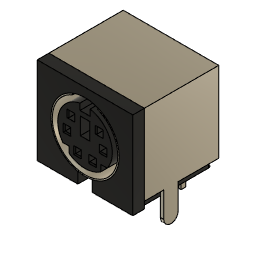
CUI_MD-60SM (Autodesk Fusion 360 design; units mm, degrees)
Autodesk Fusion 360 part; units mm, degrees
note: some values were not read from the file. Set by a fixed rule: which sketch regions a step uses.
sketch "Sketch1" plane through (0, 0, 0) normal (0, 1, 0) x (1, 0, 0) in component "Front"
  line L0 (-7, 0) -> (7, 0)
  line L1 (7, 0) -> (7, -12.8)
  line L2 (7, -12.8) -> (-7, -12.8)
  line L3 (-7, -12.8) -> (-7, 0)
  circle A0 centre (0, -6.5) radius 5
  line L4 (0, 0) -> (0, -12.8) construction
  dimension "d2" = 14
  dimension "d3" = 12.8
  dimension "d4" = 10
  dimension "d5" = 6.5
  constraint horizontal L0
  constraint vertical L1
  constraint horizontal L2
  constraint vertical L3
  constraint midpoint L4.start L0
  constraint coincident L4.start origin
  constraint midpoint L2 L4.end
  constraint coincident A0.centre L4
  measures "d2" distance of L0.start L0.end
  measures "d3" distance of L0.start L2.end
  measures "d4" diameter of A0
  measures "d5" distance of L4.start A0.centre
extrude "Extrude1" add sketch "Sketch1" along normal blind 1.7 makes body 1 in component "Front"
sketch "Sketch1 (2)" plane through (0, 1.7, 0) normal (0, 1, 0) x (-1, 0, 0) in component "Base"
  circle A0 centre (0, 6.5) radius 5
  line L0 (7, 12.8) -> (-7, 12.8)
  line L1 (-7, 12.8) -> (-7, 0)
  line L2 (-7, 0) -> (7, 0)
  line L3 (7, 0) -> (7, 12.8)
  line L4 (-6.5, 0) -> (6.5, 0)
  line L5 (6.5, 0) -> (6.5, 3.6)
  line L6 (6.5, 3.6) -> (-6.5, 3.6)
  line L7 (-6.5, 3.6) -> (-6.5, 0)
  dimension "d8" = 3.6
  dimension "d13" = 0.5
  constraint horizontal L4
  constraint vertical L5
  constraint horizontal L6
  constraint vertical L7
  constraint coincident L4.start L7.end
  constraint coincident L5.end L6.start
  constraint coincident L4.end L5.start
  constraint midpoint origin L4
  measures "d8" distance of L4.end L5.end
  measures "d13" distance of L1.end L4.start
extrude "Extrude1'" add sketch "Sketch1 (2)" along normal blind 10.4 separate body contours A0 L6 | A0 L2 L4 L5 L6 L7 picked at (-1.2021, 3.4122) makes body 2 in component "Base"
sketch "Sketch2" plane through (0, 1.7, 0) normal (0, -1, 0) x (1, 0, 0) in component "Base"
  line L0 (6.5, 0) -> (6.5, 3.6)
  line L1 (6.5, 3.6) -> (-6.5, 3.6)
  line L2 (-6.5, 3.6) -> (-6.5, 0)
  line L3 (-6.5, 0) -> (6.5, 0)
  circle A0 centre (0, 6.5) radius 5
extrude "Extrude2" cut sketch "Sketch2" against normal blind 3.3 contours L1 A0 | L1 A0 bodies 2 in component "Base"
fillet "Fillet1" radius 0.5 2 edges at (6.5, 12.1, 1.8) (-6.5, 12.1, 1.8) on bodies 2 in component "Base"
sketch "Sketch3" plane through (0, 0, 3.6) normal (0, 0, 1) x (-1, 0, 0) in component "Base"
  arc A0 (6, -12.1) -> (6.5, -11.6) centre (6, -11.6) ccw
  line L0 (6.5, -11.6) -> (6.5, -1.7)
  line L1 (6.5, -1.7) -> (4.0731, -1.7)
  line L2 (4.0731, -1.7) -> (4.0731, -5)
  line L3 (4.0731, -5) -> (-4.0731, -5)
  line L4 (-4.0731, -5) -> (-4.0731, -1.7)
  line L5 (-4.0731, -1.7) -> (-6.5, -1.7)
  line L6 (-6.5, -1.7) -> (-6.5, -11.6)
  arc A1 (-6.5, -11.6) -> (-6, -12.1) centre (-6, -11.6) ccw
  line L7 (-6, -12.1) -> (6, -12.1)
  line L8 (6.5, -5) -> (-6.5, -5)
  line L9 (-6.5, -5) -> (-6.5, -7)
  line L10 (-6.5, -7) -> (6.5, -7)
  line L11 (6.5, -7) -> (6.5, -5)
  dimension "d16" = 2
  constraint horizontal L8
  constraint vertical L9
  constraint horizontal L10
  constraint vertical L11
  constraint coincident L0 L8.start
  constraint collinear L6 L9
  constraint coincident L3.end L8
  measures "d16" distance of L8.start L10.end
extrude "Extrude3" add sketch "Sketch3" along normal up to surface (8.7 mm away) contours L0 L3 L6 L8 L9 L10 L11 bodies 2 in component "Base"
sketch "Sketch1 (3)" plane through (0, 5, 0) normal (0, -1, 0) x (1, 0, 0) in component "Jack"
  arc A0 (-4.0731, 3.6) -> (4.0731, 3.6) centre (0, 6.5) ccw
  line L0 (4.0731, 3.6) -> (6.5, 3.6)
  line L1 (6.5, 3.6) -> (6.5, 12.3)
  line L2 (6.5, 12.3) -> (-6.5, 12.3)
  line L3 (-6.5, 12.3) -> (-6.5, 3.6)
  line L4 (-6.5, 3.6) -> (-4.0731, 3.6)
  circle A1 centre (0, 6.5) radius 5
  circle A2 centre (0, 6.5) radius 4 construction
  line L5 (-0.75, 10.4291) -> (-0.75, 9.5)
  line L6 (-0.75, 9.5) -> (0.75, 9.5)
  line L7 (0.75, 9.5) -> (0.75, 10.4291)
  line L8 (0, 12.3) -> (0, 0) construction
  line L9 (-3.2524, 4.1716) -> (-2.3284, 4.1716)
  line L10 (-2.3284, 4.1716) -> (-2.3284, 3.2476)
  line L11 (3.2524, 4.1716) -> (2.3284, 4.1716)
  line L12 (2.3284, 4.1716) -> (2.3284, 3.2476)
  arc A3 (-0.75, 10.4291) -> (-3.2524, 4.1716) centre (0, 6.5) ccw
  arc A4 (3.2524, 4.1716) -> (0.75, 10.4291) centre (0, 6.5) ccw
  arc A5 (-2.3284, 3.2476) -> (2.3284, 3.2476) centre (0, 6.5) ccw
  dimension "d19" = 8
  dimension "d20" = 1.5
  dimension "d21" = 0.9291
  dimension "d22" = 0.924
  constraint concentric A0 A2
  constraint coincident A2 L5.start
  constraint vertical L5
  constraint perpendicular L5 L6
  constraint coincident A2 L7.end
  constraint perpendicular L6 L7
  constraint midpoint L2 L8.start
  constraint coincident L8.end origin
  constraint symmetric L5.end L6.end L8
  constraint coincident A2 L9.start
  constraint horizontal L9
  constraint coincident A2 L10.end
  constraint perpendicular L9 L10
  constraint coincident A2 L11.start
  constraint perpendicular L10 L11
  constraint coincident A2 L12.end
  constraint perpendicular L11 L12
  constraint equal L9 L10
  constraint equal L10 L11
  constraint equal L11 L12
  constraint concentric A2 A3
  constraint coincident A0.centre A1.centre
  constraint concentric A2 A4
  measures "d19" diameter of A2
  measures "d20" distance of L5.end L6.end
  measures "d21" distance of L6.end L7.end
  measures "d22" distance of L9.start L9.end
extrude "Extrude1''" add sketch "Sketch1 (3)" along normal up to surface (5 mm away) separate body contours L5 L6 L7 L9 L10 L11 L12 A3 A4 A5 makes body 3 in component "Jack"
sketch "Sketch2 (2)" plane through (0, 0, 0) normal (0, -1, 0) x (1, 0, 0) in component "Jack"
  line L0 (-0.75, 9.5) -> (-0.75, 10.4291)
  arc A0 (-0.75, 10.4291) -> (-3.2524, 4.1716) centre (0, 6.5) ccw
  line L1 (-3.2524, 4.1716) -> (-2.3284, 4.1716)
  line L2 (-2.3284, 4.1716) -> (-2.3284, 3.2476)
  arc A1 (-2.3284, 3.2476) -> (2.3284, 3.2476) centre (0, 6.5) ccw
  line L3 (2.3284, 3.2476) -> (2.3284, 4.1716)
  line L4 (2.3284, 4.1716) -> (3.2524, 4.1716)
  arc A2 (3.2524, 4.1716) -> (0.75, 10.4291) centre (0, 6.5) ccw
  line L5 (0.75, 10.4291) -> (0.75, 9.5)
  line L6 (0.75, 9.5) -> (-0.75, 9.5)
  circle A3 centre (0, 6.5) radius 4 construction
  line L7 (0, 0) -> (0, 12.3) construction
  line L8 (-4, 6.5) -> (4, 6.5) construction
  line L9 (-2.5, 8.585) -> (-1.65, 8.585)
  line L10 (-1.65, 8.585) -> (-1.65, 7.635)
  line L11 (-1.65, 7.635) -> (-2.5, 7.635)
  line L12 (-2.5, 7.635) -> (-2.5, 8.585)
  line L13 (1.65, 8.585) -> (2.5, 8.585)
  line L14 (2.5, 8.585) -> (2.5, 7.635)
  line L15 (2.5, 7.635) -> (1.65, 7.635)
  line L16 (1.65, 7.635) -> (1.65, 8.585)
  line L17 (-3.055, 6.515) -> (-2.105, 6.515)
  line L18 (-2.105, 6.515) -> (-2.105, 5.665)
  line L19 (-2.105, 5.665) -> (-3.055, 5.665)
  line L20 (-3.055, 5.665) -> (-3.055, 6.515)
  line L21 (2.105, 6.515) -> (3.055, 6.515)
  line L22 (3.055, 6.515) -> (3.055, 5.665)
  line L23 (3.055, 5.665) -> (2.105, 5.665)
  line L24 (2.105, 5.665) -> (2.105, 6.515)
  line L25 (-1.51, 4.435) -> (-0.56, 4.435)
  line L26 (-0.56, 4.435) -> (-0.56, 3.585)
  line L27 (-0.56, 3.585) -> (-1.51, 3.585)
  line L28 (-1.51, 3.585) -> (-1.51, 4.435)
  line L29 (0.56, 4.435) -> (1.51, 4.435)
  line L30 (1.51, 4.435) -> (1.51, 3.585)
  line L31 (1.51, 3.585) -> (0.56, 3.585)
  line L32 (0.56, 3.585) -> (0.56, 4.435)
  line L33 (2.105, 6.515) -> (3.055, 5.665) construction
  line L34 (3.055, 6.515) -> (2.105, 5.665) construction
  line L35 (1.65, 8.585) -> (2.5, 7.635) construction
  line L36 (2.5, 8.585) -> (1.65, 7.635) construction
  line L37 (-2.5, 8.585) -> (-1.65, 7.635) construction
  line L38 (-1.65, 8.585) -> (-2.5, 7.635) construction
  line L39 (-3.055, 6.515) -> (-2.105, 5.665) construction
  line L40 (-2.105, 6.515) -> (-3.055, 5.665) construction
  line L41 (-1.51, 4.435) -> (-0.56, 3.585) construction
  line L42 (-0.56, 4.435) -> (-0.4693, 4.435)
  line L43 (-1.51, 3.585) -> (-0.56, 4.435) construction
  line L44 (0.56, 4.435) -> (1.51, 3.585) construction
  line L45 (1.51, 4.435) -> (0.56, 3.585) construction
  line L46 (-2.075, 8.585) -> (-2.075, 7.635) construction
  line L47 (2.075, 8.585) -> (2.075, 7.635) construction
  line L48 (-2.075, 8.11) -> (2.075, 8.11) construction
  line L49 (-2.58, 6.515) -> (-2.58, 6.4)
  line L50 (-2.58, 6.4) -> (-2.58, 5.665) construction
  line L51 (2.58, 6.515) -> (2.58, 5.665) construction
  line L52 (-2.58, 6.09) -> (2.58, 6.09) construction
  line L53 (-1.035, 4.01) -> (1.035, 4.01) construction
  line L54 (0.69, 6.32) -> (-0.69, 6.32)
  line L55 (-0.69, 6.32) -> (-0.69, 8.81)
  line L56 (-0.69, 8.81) -> (0.69, 8.81)
  line L57 (0.69, 8.81) -> (0.69, 6.32)
  line L58 (0.69, 6.32) -> (-0.69, 8.81) construction
  line L59 (-0.69, 6.32) -> (0.69, 8.81) construction
  point P0 (0, 7.565)
  dimension "d27" = 0.85
  dimension "d28" = 0.95
  dimension "d29" = 0.85
  dimension "d30" = 0.95
  dimension "d43" = 5.16
  dimension "d48" = 8
  dimension "d49" = 4.15
  dimension "d50" = 2.07
  dimension "d51" = 1.61
  dimension "d52" = 0.41
  dimension "d53" = 2.49
  dimension "d54" = 1.38
  dimension "d55" = 2.49
  dimension "d56" = 2.31
  constraint tangent A0 A3
  constraint concentric A2 A3
  constraint coincident L7.start origin
  constraint vertical L7
  constraint coincident A3 L8.start
  constraint coincident A2 L8.end
  constraint coincident A0.centre L8
  constraint horizontal L8
  constraint horizontal L9
  constraint vertical L10
  constraint horizontal L11
  constraint vertical L12
  constraint horizontal L13
  constraint vertical L14
  constraint horizontal L15
  constraint vertical L16
  constraint horizontal L17
  constraint vertical L18
  constraint horizontal L19
  constraint vertical L20
  constraint horizontal L21
  constraint vertical L22
  constraint horizontal L23
  constraint vertical L24
  constraint horizontal L25
  constraint vertical L26
  constraint horizontal L27
  constraint vertical L28
  constraint horizontal L29
  constraint vertical L30
  constraint horizontal L31
  constraint vertical L32
  constraint equal L25 L29
  constraint equal L28 L32
  constraint equal L17 L25
  constraint equal L17 L21
  constraint equal L20 L28
  constraint equal L20 L24
  constraint equal L9 L13
  constraint equal L12 L16
  constraint collinear L19 L23
  constraint collinear L27 L31
  constraint coincident L25 L42.end
  constraint midpoint L9 L46.start
  constraint midpoint L11 L46.end
  constraint midpoint L13 L47.start
  constraint midpoint L15 L47.end
  constraint midpoint L46 L48.start
  constraint midpoint L36 L48.end
  constraint perpendicular L47 L48
  constraint symmetric L7 L48.start L48.end
  constraint midpoint L17 L49.start
  constraint perpendicular L17 L49
  constraint midpoint L19 L50.end
  constraint perpendicular L19 L50
  constraint midpoint L21 L51.start
  constraint midpoint L23 L51.end
  constraint midpoint L39 L52.start
  constraint midpoint L51 L52.end
  constraint perpendicular L51 L52
  constraint symmetric L7 L52.start L52.end
  constraint midpoint L41 L53.start
  constraint midpoint L44 L53.end
  constraint symmetric L7 L53.start L53.end
  constraint horizontal L54
  constraint perpendicular L54 L55
  constraint parallel L54 L56
  constraint parallel L55 L57
  constraint coincident L58 P0
  constraint coincident L59 P0
  constraint coincident L7 P0
  measures "d27" distance of L25.start L27.end
  measures "d28" distance of L25.start L25.end
  measures "d29" distance of L9.start L9.end
  measures "d30" distance of L9.start L11.end
  measures "d43" distance of L52.start L52.end
  measures "d48" diameter of A3
  measures "d49" distance of L48.start L48.end
  measures "d50" distance of L53.start L53.end
  measures "d51" distance of L8 L48
  measures "d52" distance of L8 L52
  measures "d53" distance of L8 L53
  measures "d54" distance of L55.end L56.end
  measures "d55" distance of L54.end L55.end
  measures "d56" distance of L8 L56.end
extrude "Extrude2'" cut sketch "Sketch2 (2)" against normal blind 5 contours L9 L10 L11 L12 | L13 L14 L15 L16 | L17 L18 L19 L20 | L21 L22 L23 L24 | L25 L26 L27 L28 | L29 L30 L31 L32 | L54 L55 L56 L57 bodies 3 in component "Jack"
chamfer "Chamfer1" distance 0.15 angle 45 18 edges at (-2.5, 0, 8.11) (-2.075, 0, 8.585) (-1.65, 0, 8.11) (1.65, 0, 8.11) (2.075, 0, 8.585) (2.5, 0, 8.11) (-2.58, 0, 6.515) (-3.055, 0, 6.09) (-2.58, 0, 5.665) (-1.035, 0, 4.435) (-1.51, 0, 4.01) (-1.035, 0, 3.585) (1.035, 0, 3.585) (1.51, 0, 4.01) (1.035, 0, 4.435) (2.58, 0, 5.665) (3.055, 0, 6.09) (2.58, 0, 6.515) on bodies 3 in component "Jack"
sketch "Sketch1 (4)" plane through (0, 5, 0) normal (0, -1, 0) x (1, 0, 0) in component "Barrel"
  arc A0 (-4.0731, 3.6) -> (4.0731, 3.6) centre (0, 6.5) ccw
  line L0 (4.0731, 3.6) -> (6.5, 3.6)
  line L1 (6.5, 3.6) -> (6.5, 12.3)
  line L2 (6.5, 12.3) -> (-6.5, 12.3)
  line L3 (-6.5, 12.3) -> (-6.5, 3.6)
  line L4 (-6.5, 3.6) -> (-4.0731, 3.6)
  circle A1 centre (0, 6.5) radius 5
  arc A2 (-1.9134, 11.1194) -> (1.9134, 11.1194) centre (0, 6.5) ccw
  line L5 (0, 6.5) -> (-1.9134, 11.1194) construction
  line L6 (0, 6.5) -> (1.9134, 11.1194) construction
  line L7 (0, 6.5) -> (0, 12.3) construction
  arc A3 (-1.8369, 10.9346) -> (1.8369, 10.9346) centre (0, 6.5) ccw
  line L8 (1.8369, 10.9346) -> (1.9134, 11.1194)
  line L9 (-1.8369, 10.9346) -> (-1.9134, 11.1194)
  dimension "d58" = 315
  dimension "d60" = 0.2
  constraint coincident A1 A2.start
  constraint coincident A0.centre A1.centre
  constraint midpoint L2 L7.end
  constraint symmetric A2.start A2.end L7
  constraint coincident L5 A3.start
  constraint parallel L6 L8
  measures "d60" distance of A2.end A3.end
extrude "Extrude1'''" add sketch "Sketch1 (4)" along normal up to surface (5 mm away) separate body contours A0 A1 A2 A3 L8 L9 makes body 4 in component "Barrel"
sketch "Sketch2 (3)" plane through (0, 0, 0) normal (0, -1, 0) x (1, 0, 0) in component "Front"
  circle A0 centre (0, 6.5) radius 5
  line L0 (7, 12.8) -> (-7, 12.8)
  line L1 (-7, 12.8) -> (-7, 0)
  line L2 (-7, 0) -> (7, 0)
  line L3 (7, 0) -> (7, 12.8)
  circle A1 centre (0, 6.5) radius 5
  line L4 (-7, 0) -> (7, 0)
  line L5 (0, 0) -> (0, 6.5) construction
  line L6 (1.05, 1.6115) -> (1.05, 0)
  line L7 (-1.05, 1.6115) -> (-1.05, 0)
  line L8 (-1.05, 0) -> (1.05, 0)
  dimension "d63" = 2.1
  constraint coincident L5.start origin
  constraint coincident A0.centre A1.centre
  constraint coincident A1 L6.start
  constraint coincident L2 L6.end
  constraint perpendicular L2 L6
  constraint coincident A1 L7.start
  constraint coincident L4 L7.end
  constraint perpendicular L4 L7
  constraint symmetric L5 L6.end L7.end
  measures "d63" distance of L6.end L7.end
extrude "Extrude2''" cut sketch "Sketch2 (3)" against normal up to surface (1.7 mm away) contours A0 L2 A1 L4 L6 L7 L8 bodies 1 in component "Front"
sketch "Sketch1 (5)" plane through (0, 1.7, 0) normal (0, 1, 0) x (-1, 0, 0) in component "Shield"
  line L0 (-1.05, 0) -> (-1.05, 1.6115)
  arc A0 (1.05, 1.6115) -> (-1.05, 1.6115) centre (0, 6.5) ccw
  line L1 (1.05, 1.6115) -> (1.05, 0)
  line L2 (1.05, 0) -> (7, 0)
  line L3 (7, 0) -> (7, 12.8)
  line L4 (7, 12.8) -> (-7, 12.8)
  line L5 (-7, 12.8) -> (-7, 0)
  line L6 (-7, 0) -> (-1.05, 0)
  line L7 (-7, 12.8) -> (-7, 0)
  line L8 (7, 12.8) -> (-7, 12.8)
  line L9 (7, 0) -> (7, 12.8)
  line L10 (-6.5, 1) -> (-6.5, 12.3)
  line L11 (-6.5, 12.3) -> (6.5, 12.3)
  line L12 (6.5, 12.3) -> (6.5, 1)
  line L13 (-6.5, 1) -> (-7, 1)
  line L14 (-7, 1) -> (-7, 12.8)
  line L15 (-7, 12.8) -> (7, 12.8)
  line L16 (7, 12.8) -> (7, 1)
  line L17 (7, 1) -> (6.5, 1)
  dimension "d66" = 0.5
  dimension "d67" = 0.5
  dimension "d68" = 0.5
  dimension "d69" = 1
  dimension "d70" = 1
  constraint parallel L7 L10
  constraint perpendicular L7 L11
  constraint perpendicular L11 L12
  constraint coincident L5 L13.end
  constraint perpendicular L5 L13
  constraint coincident L4.end L5.start
  constraint coincident L3.end L4.start
  constraint coincident L9 L16.end
  constraint perpendicular L15 L16
  constraint horizontal L17
  measures "d66" distance of L4 L11
  measures "d67" distance of L5 L10
  measures "d68" distance of L9 L12
  measures "d69" vertical distance of L5.end L10.start
  measures "d70" vertical distance of L2.end L12.end
extrude "Extrude1''''" add sketch "Sketch1 (5)" along normal blind 10.4 separate body contours L3 L4 L5 L7 L8 L9 L10 L11 L12 L13 L14 L15 L16 L17 makes body 5 in component "Shield"
sketch "Sketch2 (4)" plane through (7, 0, 0) normal (1, 0, 0) x (0, 1, 0) in component "Shield"
  line L0 (1.7, 12.8) -> (1.7, 1)
  line L1 (1.7, 1) -> (12.1, 1)
  line L2 (12.1, 1) -> (12.1, 12.8)
  line L3 (12.1, 12.8) -> (1.7, 12.8)
  line L4 (0, 0) -> (0, 12.8)
  line L5 (0, 0) -> (1.7, 0)
  line L6 (1.7, 1) -> (12.1, 1)
  line L7 (4.55, 1) -> (4.55, -2.75)
  line L8 (4.55, 1) -> (6.65, 1)
  line L9 (6.65, 1) -> (6.65, -2.75)
  arc A0 (4.55, -2.75) -> (6.65, -2.75) centre (5.6, -2.75) ccw
  line L10 (5.6, 1) -> (5.6, 0.8862)
  line L11 (5.6, 0.8862) -> (5.6, -3.8) construction
  line L12 (6.65, -2.75) -> (5.6, -2.75) construction
  line L13 (5.6, -2.75) -> (4.55, -2.75) construction
  dimension "d73" = 2.1
  dimension "d74" = 180
  dimension "d75" = 3.8
  dimension "d76" = 5.6
  constraint coincident L6 L7.start
  constraint perpendicular L1 L7
  constraint coincident L6 L8.end
  constraint perpendicular L7 L8
  constraint perpendicular L6 L9
  constraint equal L7 L9
  constraint coincident L9.end A0.end
  constraint coincident L8 L10.start
  constraint perpendicular L8 L10
  constraint coincident A0 L11.end
  constraint perpendicular L8 L11
  constraint coincident A0.centre L11
  constraint coincident A0.centre L12.end
  measures "d73" distance of L7.start L8.end
  measures "d74" angle of L12 L13
  measures "d75" vertical distance of L5.end L11.end
  measures "d76" horizontal distance of L4.start L11.end
extrude "Extrude2'''" add sketch "Sketch2 (4)" against normal up to surface (0.5 mm away) contours L1 L6 L7 L8 L9 A0 bodies 5 in component "Shield"
sketch "Sketch3 (2)" plane through (-7, 0, 0) normal (-1, 0, 0) x (0, -1, 0) in component "Shield"
  line L0 (-1.7, 1) -> (-1.7, 12.8)
  line L1 (-1.7, 12.8) -> (-12.1, 12.8)
  line L2 (-12.1, 12.8) -> (-12.1, 1)
  line L3 (-12.1, 1) -> (-1.7, 1)
  line L4 (-4.55, 1) -> (-4.55, -2.75)
  line L5 (-6.65, -2.75) -> (-6.65, 1)
  arc A0 (-6.65, -2.75) -> (-4.55, -2.75) centre (-5.6, -2.75) ccw
  line L6 (-1.7, 1) -> (-12.1, 1)
extrude "Extrude3'" add sketch "Sketch3 (2)" against normal up to surface (0.5 mm away) contours L3 L4 L5 A0 L6 bodies 5 in component "Shield"
sketch "Sketch1 (6)" plane through (0, 0, 0) normal (0, 0, -1) x (1, 0, 0) in component "Pins"
  arc A0 (-6.5, -11.6) -> (-6, -12.1) centre (-6, -11.6) ccw
  line L0 (-6, -12.1) -> (6, -12.1)
  arc A1 (6, -12.1) -> (6.5, -11.6) centre (6, -11.6) ccw
  line L1 (6.5, -11.6) -> (6.5, -1.7)
  line L2 (6.5, -1.7) -> (-6.5, -1.7)
  line L3 (-6.5, -1.7) -> (-6.5, -11.6)
  line L4 (-7, 0) -> (-1.05, 0)
  line L5 (1.05, 0) -> (7, 0)
  line L6 (-7, 0) -> (7, 0) construction
  line L7 (0, 0) -> (0, -12.1) construction
  line L8 (-3.075, -8.85) -> (-3.425, -8.85)
  line L9 (-3.425, -8.85) -> (-3.425, -8.15)
  line L10 (-3.425, -8.15) -> (-3.075, -8.15)
  line L11 (-3.075, -8.15) -> (-3.075, -8.85)
  line L12 (-3.075, -8.85) -> (-3.425, -8.15) construction
  line L13 (-3.425, -8.85) -> (-3.075, -8.15) construction
  line L14 (-1.075, -8.85) -> (-1.425, -8.85)
  line L15 (-1.425, -8.85) -> (-1.425, -8.15)
  line L16 (-1.425, -8.15) -> (-1.075, -8.15)
  line L17 (-1.075, -8.15) -> (-1.075, -8.85)
  line L18 (-1.075, -8.85) -> (-1.425, -8.15) construction
  line L19 (-1.425, -8.85) -> (-1.075, -8.15) construction
  line L20 (1.425, -8.85) -> (1.075, -8.85)
  line L21 (1.075, -8.85) -> (1.075, -8.15)
  line L22 (1.075, -8.15) -> (1.425, -8.15)
  line L23 (1.425, -8.15) -> (1.425, -8.85)
  line L24 (1.425, -8.85) -> (1.075, -8.15) construction
  line L25 (1.075, -8.85) -> (1.425, -8.15) construction
  line L26 (3.425, -8.85) -> (3.075, -8.85)
  line L27 (3.075, -8.85) -> (3.075, -8.15)
  line L28 (3.075, -8.15) -> (3.425, -8.15)
  line L29 (3.425, -8.15) -> (3.425, -8.85)
  line L30 (3.425, -8.85) -> (3.075, -8.15) construction
  line L31 (3.075, -8.85) -> (3.425, -8.15) construction
  line L32 (-3.075, -11.35) -> (-3.425, -11.35)
  line L33 (-3.425, -11.35) -> (-3.425, -10.65)
  line L34 (-3.425, -10.65) -> (-3.075, -10.65)
  line L35 (-3.075, -10.65) -> (-3.075, -11.35)
  line L36 (-3.075, -11.35) -> (-3.425, -10.65) construction
  line L37 (-3.425, -11.35) -> (-3.075, -10.65) construction
  line L38 (3.425, -11.35) -> (3.075, -11.35)
  line L39 (3.075, -11.35) -> (3.075, -10.65)
  line L40 (3.075, -10.65) -> (3.425, -10.65)
  line L41 (3.425, -10.65) -> (3.425, -11.35)
  line L42 (3.425, -11.35) -> (3.075, -10.65) construction
  line L43 (3.075, -11.35) -> (3.425, -10.65) construction
  line L44 (-3.25, -11) -> (3.25, -11) construction
  line L45 (-3.25, -8.5) -> (3.25, -8.5) construction
  point P0 (-3.25, -8.5)
  point P1 (-1.25, -8.5)
  point P2 (1.25, -8.5)
  point P3 (3.25, -8.5)
  point P4 (-3.25, -11)
  point P5 (3.25, -11)
  dimension "d32" = 1.525
  dimension "d81" = 0.7
  dimension "d82" = 0.35
  dimension "d83" = 6.5
  dimension "d84" = 2.5
  dimension "d85" = 6.5
  dimension "d86" = 2.5
  dimension "d87" = 8.5
  constraint coincident L4.start L6.start
  constraint coincident L5.end L6.end
  constraint coincident L7.start origin
  constraint midpoint L0 L7.end
  constraint horizontal L8
  constraint perpendicular L8 L9
  constraint parallel L8 L10
  constraint parallel L9 L11
  constraint coincident L12 P0
  constraint coincident L13 P0
  constraint horizontal L14
  constraint perpendicular L14 L15
  constraint parallel L14 L16
  constraint parallel L15 L17
  constraint coincident L18 P1
  constraint coincident L19 P1
  constraint horizontal L20
  constraint perpendicular L20 L21
  constraint parallel L20 L22
  constraint parallel L21 L23
  constraint coincident L24 P2
  constraint coincident L25 P2
  constraint horizontal L26
  constraint perpendicular L26 L27
  constraint parallel L26 L28
  constraint parallel L27 L29
  constraint coincident L30 P3
  constraint coincident L31 P3
  constraint horizontal L32
  constraint perpendicular L32 L33
  constraint parallel L32 L34
  constraint parallel L33 L35
  constraint coincident L36 P4
  constraint coincident L37 P4
  constraint horizontal L38
  constraint perpendicular L38 L39
  constraint parallel L38 L40
  constraint parallel L39 L41
  constraint coincident L42 P5
  constraint coincident L43 P5
  constraint equal L10 L16
  constraint equal L16 L22
  constraint equal L22 L28
  constraint equal L28 L40
  constraint equal L34 L40
  constraint equal L9 L15
  constraint equal L15 L21
  constraint equal L21 L27
  constraint equal L27 L39
  constraint equal L33 L39
  constraint coincident P4 L44.start
  constraint coincident P5 L44.end
  constraint horizontal L44
  constraint symmetric L7 P4 P5
  constraint coincident P0 L45.start
  constraint coincident P3 L45.end
  constraint coincident P2 L45
  constraint coincident P1 L45
  constraint horizontal L45
  constraint symmetric L7 P1 P2
  constraint symmetric L7 P0 P3
  measures "d81" distance of L8.end L9.end
  measures "d82" distance of L9.end L10.end
  measures "d83" distance of P4 P5
  measures "d84" distance of P1 P2
  measures "d85" distance of P0 P3
  measures "d86" distance of L44 L45
  measures "d87" distance of L6 L45
extrude "Extrude1'''''" add sketch "Sketch1 (6)" along normal blind 3.8 separate body contours L8 L9 L10 L11 | L14 L15 L16 L17 | L20 L21 L22 L23 | L26 L27 L28 L29 | L32 L33 L34 L35 | L38 L39 L40 L41 makes body 6 at (3.075, 8.6167, -1.2667) makes body 7 at (-3.425, 8.6167, -1.2667) makes body 8 at (3.075, 11.1167, -1.2667) makes body 9 at (1.075, 8.6167, -1.2667) makes body 10 at (-1.425, 8.6167, -1.2667) makes body 11 at (-3.425, 10.8833, -2.5333) in component "Pins"
sketch "Sketch2 (5)" plane through (0, 0, 0) normal (0, 0, -1) x (1, 0, 0) in component "Pins"
  arc A0 (-6.5, -11.6) -> (-6, -12.1) centre (-6, -11.6) ccw
  line L0 (-6, -12.1) -> (6, -12.1)
  arc A1 (6, -12.1) -> (6.5, -11.6) centre (6, -11.6) ccw
  line L1 (6.5, -11.6) -> (6.5, -1.7)
  line L2 (6.5, -1.7) -> (-6.5, -1.7)
  line L3 (-6.5, -1.7) -> (-6.5, -11.6)
  line L4 (0, 0) -> (0, -12.1) construction
  line L5 (1.05, 0) -> (1.05, -1.7)
  line L6 (-1.05, -1.7) -> (-1.05, 0)
  line L7 (1.05, -4.875) -> (-1.05, -4.875)
  line L8 (-1.05, -4.875) -> (-1.05, -4.525)
  line L9 (-1.05, -4.525) -> (1.05, -4.525)
  line L10 (1.05, -4.525) -> (1.05, -4.875)
  line L11 (1.05, -4.875) -> (-1.05, -4.525) construction
  line L12 (-1.05, -4.875) -> (1.05, -4.525) construction
  point P0 (0, -4.7)
  dimension "d90" = 0.35
  dimension "d91" = 4.7
  constraint coincident L4.start origin
  constraint midpoint L0 L4.end
  constraint horizontal L7
  constraint perpendicular L7 L8
  constraint parallel L7 L9
  constraint parallel L8 L10
  constraint coincident L11 P0
  constraint coincident L12 P0
  constraint coincident L4 P0
  constraint collinear L5 L10
  measures "d90" distance of L7.start L9.end
  measures "d91" distance of L4.start P0
extrude "Extrude2''''" add sketch "Sketch2 (5)" along normal blind 3.8 separate body contours L7 L8 L9 L10 makes body 12 in component "Pins"
sketch "Sketch3 (3)" plane through (0, 4.525, 0) normal (0, -1, 0) x (1, 0, 0) in component "Pins"
  line L0 (1.05, 0) -> (-1.05, 0)
  line L1 (-1.05, 0) -> (-1.05, -3.8)
  line L2 (-1.05, -3.8) -> (1.05, -3.8)
  line L3 (1.05, -3.8) -> (1.05, 0)
  line L4 (0, 0) -> (0, -3.8) construction
  arc A0 (-1.05, -2.746) -> (1.05, -2.754) centre (0, -2.75) ccw
  line L5 (0, -2.75) -> (-1.05, -2.746) construction
  line L6 (0, -2.75) -> (1.05, -2.754) construction
  dimension "d94" = 180
  constraint coincident L4.start origin
  constraint midpoint L2 L4.end
  constraint coincident L1 A0.start
  constraint coincident L4 A0.centre
  constraint tangent L2 A0
  constraint tangent L3 A0
  measures "d94" angle of L5 L6
extrude "Extrude3''" cut sketch "Sketch3 (3)" against normal up to surface (0.35 mm away) contours L1 L2 A0 | L2 L3 A0 bodies 12 in component "Pins"
sketch "Sketch4" plane through (0, 12.1, 0) normal (0, 1, 0) x (-1, 0, 0) in component "Shield"
  line L0 (-6.5, 1) -> (-6.5, 12.3)
  line L1 (-6.5, 12.3) -> (6.5, 12.3)
  line L2 (6.5, 12.3) -> (6.5, 1)
  line L3 (6.5, 1) -> (7, 1)
  line L4 (7, 1) -> (7, 12.8)
  line L5 (7, 12.8) -> (-7, 12.8)
  line L6 (-7, 12.8) -> (-7, 1)
  line L7 (-7, 1) -> (-6.5, 1)
  line L8 (-7, 12.8) -> (7, 12.8)
  line L9 (7, 12.8) -> (7, 12.3)
  line L10 (7, 12.3) -> (-7, 12.3)
  line L11 (-7, 12.3) -> (-7, 12.8)
  constraint horizontal L8
  constraint vertical L9
  constraint horizontal L10
  constraint vertical L11
  constraint coincident L4 L9.end
  constraint coincident L5.end L6.start
  constraint coincident L1.end L10
extrude "Extrude4" add sketch "Sketch4" along normal blind 0.5 contours L1 L4 L5 L6 L8 L9 L10 L11 bodies 5 in component "Shield"
sketch "Sketch5" plane through (0, 0, 12.3) normal (0, 0, -1) x (1, 0, 0) in component "Shield"
  line L0 (6.5, -1.7) -> (-6.5, -1.7)
  line L1 (-6.5, -1.7) -> (-6.5, -12.1)
  line L2 (-6.5, -12.1) -> (-7, -12.1)
  line L3 (-7, -12.1) -> (-7, -12.6)
  line L4 (-7, -12.6) -> (7, -12.6)
  line L5 (7, -12.6) -> (7, -12.1)
  line L6 (7, -12.1) -> (6.5, -12.1)
  line L7 (6.5, -12.1) -> (6.5, -1.7)
  line L8 (-7, -12.6) -> (7, -12.6)
  line L9 (7, -12.6) -> (7, -12.1)
  line L10 (7, -12.1) -> (-7, -12.1)
  line L11 (-7, -12.1) -> (-7, -12.6)
  constraint horizontal L8
  constraint vertical L9
  constraint horizontal L10
  constraint vertical L11
  constraint coincident L5.end L6.start
  constraint coincident L3.end L4.start
extrude "Extrude5" add sketch "Sketch5" along normal up to surface (11.3 mm away) contours L2 L3 L4 L5 L6 L8 L9 L10 L11 bodies 5 in component "Shield"
component "Front" placed x (1, 0, 0) y (0, 1, 0) z (0, 0, 1) at (0, 0, 0)
component "Base" placed x (1, 0, 0) y (0, 1, 0) z (0, 0, 1) at (0, 0, 0)
component "Shield" placed x (1, 0, 0) y (0, 1, 0) z (0, 0, 1) at (0, 0, 0)
component "Jack" placed x (1, 0, 0) y (0, 1, 0) z (0, 0, 1) at (0, 0, 0)
component "Barrel" placed x (1, 0, 0) y (0, 1, 0) z (0, 0, 1) at (0, 0, 0)
component "Pins" placed x (1, 0, 0) y (0, 1, 0) z (0, 0, 1) at (0, 0, 0)
equation "d67 = d66"
equation "d68 = d66"
equation "d70 = d69"
